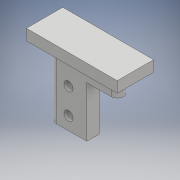
# Autodesk Inventor part: StartSupport
Saved by Autodesk Inventor 2018 (Build 220112000, 112)
## iProperties
Created: 2020-05-13
Part Number: StartSupport
Material: Generic
Document SubType Name: Modeling
Designer: Ivan
Density: 1 g/cm^3
Appearance: Default
Author: Ivan
Autodesk Inventor part; units mm, degrees
ref_plane "YZ Plane" through (0, 0, 0) normal (1, 0, 0) x (0, 1, 0)
ref_plane "XZ Plane" through (0, 0, 0) normal (0, 1, 0) x (-1, 0, 0)
ref_plane "XY Plane" through (0, 0, 0) normal (0, 0, 1) x (1, 0, 0)
sketch "Sketch1" plane through (0, 0, 0) normal (0, 0, 1) x (1, 0, 0)
  line L0 (-7.5, 1.7) -> (7.5, 1.7)
  line L1 (7.5, -1.7) -> (-7.5, -1.7)
  arc A0 (-7.5, 1.7) -> (-7.5, -1.7) centre (-7.5, 0) ccw
  arc A1 (7.5, -1.7) -> (7.5, 1.7) centre (7.5, 0) ccw
  point P0 (0, 0)
  point P1 (0, 1.7)
  dimension "d0" = 15
  dimension "d1" = 3.4
  constraints: 4 end point, 4 point on circle, 2 centre point, 1 coincident, 1 horizontal, 1 horizontal alignment, 1 midpoint, 1 parallel, 1 vertical alignment
  measures "d0" distance of L1.start L1.end
  measures "d1" distance of L0.end L1.start
extrude "Extrusion1" add sketch "Sketch1" along normal blind 4.95
sketch "Sketch2" plane through (0, 0, 4.95) normal (0, 0, 1) x (1, 0, 0)
  line L0 (-12.5, 5) -> (12.5, 5)
  line L1 (12.5, 5) -> (12.5, -5)
  line L2 (12.5, -5) -> (-12.5, -5)
  line L3 (-12.5, -5) -> (-12.5, 5)
  point P0 (0, 0)
  point P1 (0, 5)
  point P2 (12.5, 0)
  dimension "d4" = 25
  dimension "d5" = 10
  constraints: 8 end point, 2 midpoint, 2 parallel, 1 horizontal, 1 horizontal alignment, 1 perpendicular, 1 vertical alignment
  measures "d4" distance of L1.end L2.end
  measures "d5" distance of L0.end L1.end
extrude "Extrusion2" add sketch "Sketch2" along normal blind 3
sketch "Sketch3" plane through (0, 0, 0) normal (0, 0, -1) x (-1, 0, 0)
  arc A0 (7.5, -1.7) -> (7.5, 1.7) centre (7.5, 0) ccw projected
  line L0 (-0.8, 1.7) -> (-0.8, -1.7)
  line L1 (-0.8, 1.7) -> (7.5, 1.7)
  line L2 (-0.8, -1.7) -> (7.5, -1.7)
  point P0 (0, 0)
  dimension "d8" = 10
  constraints: 6 end point, 1 horizontal
extrude "Extrusion3" add sketch "Sketch3" along normal blind 14
sketch "Sketch4" plane through (-7.5, 1.7, 4.95) normal (0, 1, 0) x (1, 0, 0)
  circle A0 centre (3.3, 8.3) radius 1.25
  circle A1 centre (3.3, 15.324) radius 1.25
  point P0 (7.5, 4.95)
  point P1 (-5, 0)
  dimension "d11" = 2.5
  dimension "d12" = 8.3
  dimension "d13" = 8.3
  dimension "d14" = 7.024
  constraints: 2 centre point, 1 equal radius, 1 vertical alignment
  measures "d11" diameter of A0
  measures "d12" horizontal distance of point (-5, 0) A0.centre
  measures "d13" horizontal distance of point (-5, 0) A0.centre
  measures "d14" distance of A0.centre A1.centre
extrude "Extrusion4" cut sketch "Sketch4" against normal through all
body "Solid1"
